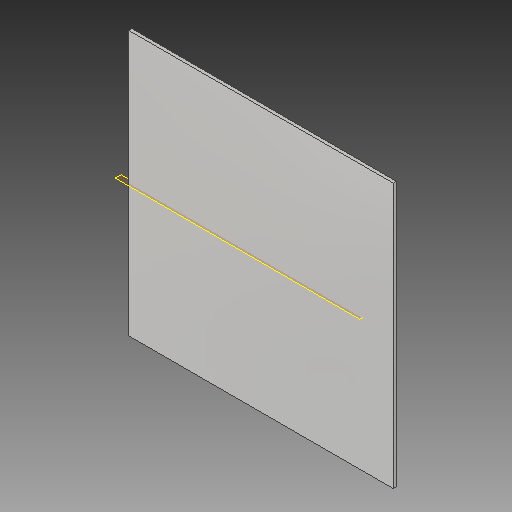
# Autodesk Inventor part: hotplate
Saved by Autodesk Inventor 2019 (Build 230136000, 136)
## iProperties
Created: 2018-10-03
Part Number: hotplate
Material: Aluminum 6061-AHC
Document SubType Name: Modeling
Designer: LillaHunden
Density: 2.7 g/cm^3
Appearance: Aluminum - Dark
Mass: 506.25 g
Surface Area: 1280 cm^2
Volume: 187.5 cm^3
Author: LillaHunden
Autodesk Inventor part; units mm, degrees
ref_plane "YZ Plane" through (0, 0, 0) normal (1, 0, 0) x (0, 1, 0)
ref_plane "XZ Plane" through (0, 0, 0) normal (0, 1, 0) x (-1, 0, 0)
ref_plane "XY Plane" through (0, 0, 0) normal (0, 0, 1) x (1, 0, 0)
sketch "Sketch1" plane through (0, 0, 0) normal (0, 0, 1) x (1, 0, 0)
  line L0 (-125, 125) -> (125, 125)
  line L1 (125, 125) -> (125, -125)
  line L2 (125, -125) -> (-125, -125)
  line L3 (-125, -125) -> (-125, 125)
  line L4 (-125, 125) -> (125, -125) construction
  line L5 (125, 125) -> (-125, -125) construction
  point P0 (0, 0)
  dimension "d0" = 250
  dimension "d1" = 250
  constraints: 12 end point, 2 midpoint, 2 parallel, 1 horizontal, 1 perpendicular
  measures "d0" distance of L1.end L2.end
  measures "d1" distance of L0.end L1.end
extrude "Extrusion1" add sketch "Sketch1" along normal blind 3
ref_plane "Work Plane1" through (-125, 0, 0) normal (0, 1, 0) x (1, 0, 0)
body "Solid1"
